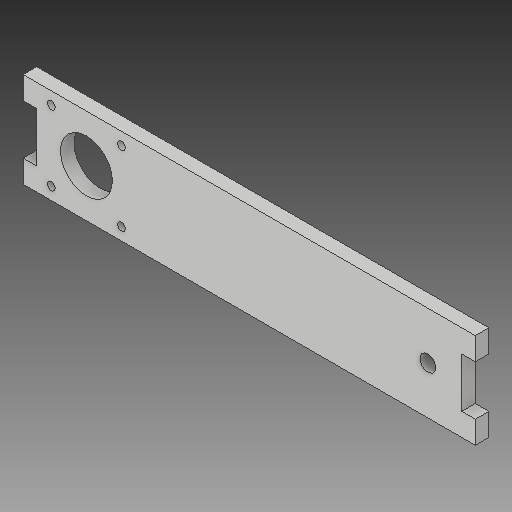
# Autodesk Inventor part: Tope riel motor
Saved by Autodesk Inventor 2019 (Build 230136000, 136)
## iProperties
Created: 2020-02-01
Part Number: Tope riel motor
Material: Generic
Document SubType Name: Modeling
Designer: Elías Sánchez
Density: 1 g/cm^3
Appearance: Default
Description: Corte Láser
Author: Elías Sánchez
Autodesk Inventor part; units mm, degrees
ref_plane "YZ Plane" through (0, 0, 0) normal (1, 0, 0) x (0, 1, 0)
ref_plane "XZ Plane" through (0, 0, 0) normal (0, 1, 0) x (-1, 0, 0)
ref_plane "XY Plane" through (0, 0, 0) normal (0, 0, 1) x (1, 0, 0)
sketch "Sketch1" plane through (0, 0, 0) normal (0, 0, 1) x (1, 0, 0)
  circle A0 centre (-15.5, 36.5) radius 1.75
  circle A1 centre (15.5, 36.5) radius 1.75
  circle A2 centre (-15.5, 5.5) radius 1.75
  circle A3 centre (15.5, 5.5) radius 1.75
  circle A4 centre (0, 21) radius 11.5
  line L0 (-28, 42) -> (172, 42)
  line L1 (172, 0) -> (-28, 0)
  line L2 (-68, 0) -> (212, 0) projected
  line L3 (-28, 42) -> (-28, 32)
  line L4 (-28, 32) -> (-22, 32)
  line L5 (-22, 32) -> (-22, 10)
  line L6 (-22, 10) -> (-28, 10)
  line L7 (-28, 10) -> (-28, 0)
  line L8 (172, 42) -> (172, 32)
  line L9 (172, 32) -> (166, 32)
  line L10 (166, 32) -> (166, 10)
  line L11 (166, 10) -> (172, 10)
  line L12 (172, 10) -> (172, 0)
  circle A5 centre (151, 21) radius 3.5
  point P0 (0, 0)
  point P1 (0, 0)
  dimension "d13" = 3.5
  dimension "d14" = 3.5
  dimension "d15" = 15.5
  dimension "d16" = 15.5
  dimension "d21" = 3.5
  dimension "d22" = 3.5
  dimension "d23" = 31
  dimension "d24" = 23
  dimension "d29" = 21
  dimension "d30" = 15.5
  dimension "d31" = 200
  dimension "d32" = 21
  dimension "d34" = 21
  dimension "d35" = 6
  dimension "d36" = 10
  dimension "d37" = 10
  dimension "d38" = 28
  dimension "d39" = 10
  dimension "d40" = 10
  dimension "d41" = 6
  dimension "d42" = 7
  dimension "d43" = 15
  dimension "d44" = 21
  constraints: 24 end point, 8 perpendicular, 6 centre point, 3 vertical alignment, 2 coincident, 2 horizontal alignment, 2 point on line, 2 vertical, 1 horizontal, 1 parallel
  measures "d13" diameter of A0
  measures "d14" diameter of A1
  measures "d15" horizontal distance of point (0, 0) A0.centre
  measures "d16" horizontal distance of point (0, 0) A1.centre
  measures "d21" diameter of A2
  measures "d22" diameter of A3
  measures "d23" distance of A3.centre A1.centre
  measures "d24" diameter of A4
  measures "d29" distance from line of L0 A4.centre
  measures "d30" horizontal distance of A0.centre A4.centre
  measures "d31" distance of L0.start L0.end
  measures "d32" distance from line of A4.centre L1
  measures "d34" distance from line of L2 A4.centre
  measures "d35" distance of L5.end L6.end
  measures "d36" distance between parallel lines of L2 L6
  measures "d37" distance between parallel lines of L0 L4
  measures "d38" distance from line of point (0, 0) L7
  measures "d39" distance of L0.end L8.end
  measures "d40" distance of L11.end L1.start
  measures "d41" distance of L8.end L9.end
  measures "d42" diameter of A5
  measures "d43" distance from line of L10 A5.centre
  measures "d44" distance from line of L1 A5.centre
extrude "Extrusion2" add sketch "Sketch1" along normal blind 6
equation "\"d14\" = d13"
equation "\"d16\" = d15"
equation "\"d21\" = d13"
equation "\"d22\" = d13"
equation "\"d37\" = d36"
equation "\"d39\" = d36"
equation "\"d40\" = d39"
equation "\"d41\" = d35"
body "Solid2"
